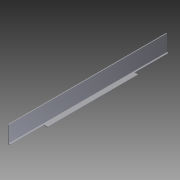
# Autodesk Inventor part: frame 7 outside L
Saved by Autodesk Inventor 2012 (Build 160160000, 160)
## iProperties
Created: 2013-08-24
Part Number: frame 7 outside L
Material: Default
Document SubType Name: Modeling
Designer: Bryce
Density: 1 g/cm^3
Author: Bryce
Autodesk Inventor part; units mm, degrees
ref_plane "YZ Plane" through (0, 0, 0) normal (1, 0, 0) x (0, 1, 0)
ref_plane "XZ Plane" through (0, 0, 0) normal (0, 1, 0) x (-1, 0, 0)
ref_plane "XY Plane" through (0, 0, 0) normal (0, 0, 1) x (1, 0, 0)
sketch "Sketch1" plane through (0, 0, 0) normal (0, 0, 1) x (1, 0, 0)
  line L0 (0, 0) -> (25.4, 0)
  line L1 (25.4, 0) -> (25.4, 3.175)
  line L2 (3.175, 76.2) -> (0, 76.2)
  line L3 (0, 76.2) -> (0, 0)
  line L4 (3.175, 76.2) -> (3.175, 3.175)
  line L5 (3.175, 3.175) -> (25.4, 3.175)
  dimension "d0" = 76.2
  dimension "d1" = 25.4
  dimension "d2" = 3.175
  dimension "d3" = 3.175
  constraints: 12 end point, 2 parallel, 1 horizontal, 1 perpendicular
  measures "d0" distance of L2.end L0.start
  measures "d1" distance of L0.start L0.end
  measures "d2" distance between parallel lines of L0 L5
  measures "d3" distance between parallel lines of L3 L4
extrude "Extrusion1" add sketch "Sketch1" along normal blind 711.2
sketch "Sketch2" plane through (0, 0, 0) normal (0, -1, 0) x (1, 0, 0)
  line L0 (0, 0) -> (0, 711.2) projected
  line L1 (25.4, 0) -> (25.4, 711.2) projected
  line L2 (0, 355.6) -> (25.4, 355.6)
  line L3 (25.4, 0) -> (9.525, 0)
  line L4 (9.525, 0) -> (9.525, 152.4)
  line L5 (9.525, 152.4) -> (25.4, 152.4)
  line L6 (25.4, 152.4) -> (25.4, 0)
  line L7 (25.4, 711.2) -> (9.525, 711.2)
  line L8 (9.525, 711.2) -> (9.525, 558.8)
  line L9 (9.525, 558.8) -> (25.4, 558.8)
  line L10 (25.4, 558.8) -> (25.4, 711.2)
  dimension "d7" = 15.875
  dimension "d8" = 152.4
  constraints: 18 end point, 3 symmetric about line, 2 midpoint, 2 parallel, 1 horizontal, 1 perpendicular
  measures "d7" distance of L1.start L3.end
  measures "d8" distance of L1.start L5.end
extrude "Extrusion2" cut sketch "Sketch2" against normal through all
equation "\"d3\" = d2"
body "Solid1"
